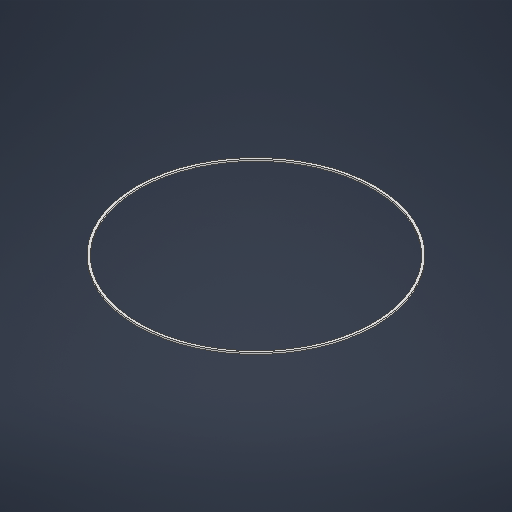
# Autodesk Inventor part: camera_base_test_print
Saved by Autodesk Inventor 2026.2 (Build 302298000, 298)
## iProperties
Created: 2026-02-25
Part Number: camera_base_test_print
Material: Generic
Document SubType Name: Modeling
Designer: Tathagata Sikdar
Density: 1 g/cm^3
Appearance: Default
Author: Tathagata Sikdar
Autodesk Inventor part; units mm, degrees
ref_plane "YZ Plane" through (0, 0, 0) normal (1, 0, 0) x (0, 1, 0)
ref_plane "XZ Plane" through (0, 0, 0) normal (0, 1, 0) x (-1, 0, 0)
ref_plane "XY Plane" through (0, 0, 0) normal (0, 0, 1) x (1, 0, 0)
sketch "Sketch1" plane through (0, 0, 0) normal (0, 1, 0) x (-1, 0, 0)
  line L0 (0, -60.0444) -> (52, 30.0222) construction
  line L1 (52, 30.0222) -> (-52, 30.0222) construction
  line L2 (-52, 30.0222) -> (0, -60.0444) construction
  line L3 (-26, -15.0111) -> (52, 30.0222) construction
  line L4 (0, -60.0444) -> (0, 30.0222) construction
  circle A0 centre (0, -60.0444) radius 2
  circle A1 centre (-52, 30.0222) radius 2
  circle A2 centre (52, 30.0222) radius 2
  circle A3 centre (0, 0) radius 69.5444
  line L5 (87.0538, 1.5094) -> (87.0538, 83.0538)
  line L6 (-87.0538, 1.5094) -> (-87.0538, 83.0538)
  line L7 (83.0538, 87.0538) -> (-83.0538, 87.0538)
  circle A4 centre (52, 30.0222) radius 5.75
  circle A5 centre (52, 30.0222) radius 3.75
  circle A6 centre (-52, 30.0222) radius 3.75
  circle A7 centre (-52, 30.0222) radius 5.75
  circle A8 centre (0, -60.0444) radius 3.75
  circle A9 centre (0, -60.0444) radius 5.75
  circle A10 centre (-83.0538, 83.0538) radius 2
  circle A11 centre (83.0538, 83.0538) radius 2
  circle A12 centre (0, -81.5444) radius 2
  arc A13 (-87.0538, 1.5094) -> (87.0538, 1.5094) centre (0, 1.5094) ccw
  line L8 (85.6338, 1.5094) -> (85.6338, 76.6475)
  arc A14 (79.6411, 82.8301) -> (82.8301, 79.6411) centre (83.0538, 83.0538) ccw
  line L9 (76.6475, 85.6338) -> (-76.6475, 85.6338)
  arc A15 (-82.8301, 79.6411) -> (-79.6411, 82.8301) centre (-83.0538, 83.0538) ccw
  line L10 (-85.6338, 76.6475) -> (-85.6338, 1.5094)
  arc A16 (3.4015, -81.1891) -> (-3.4015, -81.1891) centre (0, -81.5444) ccw
  arc A17 (-82.8301, 79.6411) -> (-85.6338, 76.6475) centre (-82.6338, 76.6475) ccw
  arc A18 (-76.6475, 85.6338) -> (-79.6411, 82.8301) centre (-76.6475, 82.6338) ccw
  arc A19 (79.6411, 82.8301) -> (76.6475, 85.6338) centre (76.6475, 82.6338) ccw
  arc A20 (85.6338, 76.6475) -> (82.8301, 79.6411) centre (82.6338, 76.6475) ccw
  arc A21 (6.6171, -83.8684) -> (85.6338, 1.5094) centre (0, 1.5094) ccw
  arc A22 (-85.6338, 1.5094) -> (-6.6171, -83.8684) centre (0, 1.5094) ccw
  line L11 (81.4738, 1.5094) -> (81.4738, 74.8709)
  arc A23 (75.8246, 80.7745) -> (80.7745, 75.8246) centre (83.0538, 83.0538) ccw
  line L12 (74.8709, 81.4738) -> (-74.8709, 81.4738)
  arc A24 (-80.7745, 75.8246) -> (-75.8246, 80.7745) centre (-83.0538, 83.0538) ccw
  line L13 (-81.4738, 74.8709) -> (-81.4738, 1.5094)
  arc A25 (-81.4738, 1.5094) -> (-8.1447, -79.5563) centre (0, 1.5094) ccw
  arc A26 (7.1071, -78.909) -> (-7.1071, -78.909) centre (0, -81.5444) ccw
  arc A27 (8.1447, -79.5563) -> (81.4738, 1.5094) centre (0, 1.5094) ccw
  arc A28 (-80.7745, 75.8246) -> (-81.4738, 74.8709) centre (-80.4738, 74.8709) ccw
  arc A29 (-74.8709, 81.4738) -> (-75.8246, 80.7745) centre (-74.8709, 80.4738) ccw
  arc A30 (75.8246, 80.7745) -> (74.8709, 81.4738) centre (74.8709, 80.4738) ccw
  arc A31 (81.4738, 74.8709) -> (80.7745, 75.8246) centre (80.4738, 74.8709) ccw
  arc A32 (7.1071, -78.909) -> (8.1447, -79.5563) centre (8.0447, -78.5613) ccw
  arc A33 (-8.1447, -79.5563) -> (-7.1071, -78.909) centre (-8.0447, -78.5613) ccw
  arc A34 (-6.6171, -83.8684) -> (-3.4015, -81.1891) centre (-6.3853, -80.8774) ccw
  arc A35 (3.4015, -81.1891) -> (6.6171, -83.8684) centre (6.3853, -80.8774) ccw
  arc A36 (87.0538, 83.0538) -> (83.0538, 87.0538) centre (83.0538, 83.0538) ccw
  arc A37 (-83.0538, 87.0538) -> (-87.0538, 83.0538) centre (-83.0538, 83.0538) ccw
  circle A38 centre (62.5538, 62.5538) radius 17.5 construction
  line L14 (-83.0538, 83.0538) -> (-87.0538, 87.0538) construction
  circle A39 centre (-85.1751, 85.1751) radius 1 construction
  circle A40 centre (62.5538, 62.5538) radius 18.92 construction
  line L15 (0, 0) -> (83.0538, 83.0538) construction
  circle A41 centre (0, 0) radius 70.9644
  arc A42 (74.5685, 80.0538) -> (80.0538, 74.5685) centre (83.0538, 83.0538) ccw
  line L16 (74.5685, 80.0538) -> (-74.5685, 80.0538)
  arc A43 (-80.0538, 74.5685) -> (-74.5685, 80.0538) centre (-83.0538, 83.0538) ccw
  line L17 (-80.0538, 74.5685) -> (-80.0538, 1.5094)
  arc A44 (-80.0538, 1.5094) -> (-8.3193, -78.111) centre (0, 1.5094) ccw
  arc A45 (8.3193, -78.111) -> (-8.3193, -78.111) centre (0, -81.5444) ccw
  arc A46 (8.3193, -78.111) -> (80.0538, 1.5094) centre (0, 1.5094) ccw
  line L18 (80.0538, 1.5094) -> (80.0538, 74.5685)
  point P0 (0, -85.5444)
  point P1 (85.6338, 85.2988)
  point P2 (80.8088, 85.6338)
  point P3 (-80.8088, 85.6338)
  point P4 (-85.6338, 80.8088)
  point P5 (0, -69.5444)
  dimension "d0" = 4
  dimension "d1" = 104
  dimension "d2" = 7.5
  dimension "d28" = 11.5
  dimension "d29" = 7.5
  dimension "d40" = 4
  dimension "d45" = 1.42
  dimension "d47" = 1.42
  dimension "d48" = 1.42
  dimension "d49" = 1.42
  dimension "d50" = 1.42
  dimension "d61" = 4.16
  dimension "d64" = 1
  dimension "d70" = 4
  dimension "d87" = 3
  dimension "d90" = 12
  dimension "ReservoirID" = 35
  dimension "d109" = 45
  dimension "d110" = 2
  dimension "d112" = 37.84
  dimension "d114" = 45
  constraints: 65 point on circle, 46 centre point, 38 end point, 36 tangent, 20 equal radius, 13 coincident, 8 point on line, 5 concentric, 4 horizontal alignment, 4 vertical alignment, 3 horizontal, 3 vertical, 2 equal length, 2 midpoint, 1 parallel, 19 other
  measures "d0" diameter of A0
  measures "d1" distance of L0.end L1.end
  measures "d28" diameter of A4
  measures "d29" diameter of A5
  measures "d40" distance of point (0, -85.544) A12.centre
  measures "d45" distance between parallel lines of L7 L9
  measures "d47" distance between parallel lines of L5 L8
  measures "d48" radial gap between concentric circles of A16 A12
  measures "d49" radial gap between concentric circles of A10 A15
  measures "d50" radial gap between concentric circles of A11 A14
  measures "d61" radial gap between concentric circles of A21 A27
  measures "d64" radius of A28
  measures "d70" radius of A36
  measures "d87" radius of A20
  measures "d90" distance of A12.centre point (0, -69.544)
  measures "ReservoirID" diameter of A38
  measures "d109" angle of L7 L14
  measures "d110" diameter of A39
  measures "d112" diameter of A40
  measures "d114" angle of L15 L4
extrude "Extrusion6" add sketch "Sketch1" along normal blind 1 contours A41
body "Solid4"
